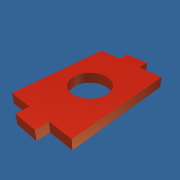
# Autodesk Inventor part: Acrylic_2.2_UpperArmBridge
Saved by Autodesk Inventor 2012 (Build 160160000, 160)
## iProperties
Created: 2014-03-29
Part Number: Acrylic_2.2_UpperArmBridge
Material: Default
Document SubType Name: Modeling
Designer: Admin
Density: 1 g/cm^3
Author: Admin
Autodesk Inventor part; units mm, degrees
ref_plane "YZ Plane" through (0, 0, 0) normal (1, 0, 0) x (0, 1, 0)
ref_plane "XZ Plane" through (0, 0, 0) normal (0, 1, 0) x (-1, 0, 0)
ref_plane "XY Plane" through (0, 0, 0) normal (0, 0, 1) x (1, 0, 0)
sketch "Sketch1" plane through (0, 0, 0) normal (0, 0, 1) x (1, 0, 0)
  line L0 (-10.5, 0) -> (10.5, 0) projected
  line L1 (0, -18.9) -> (0, 18.9) projected
  line L2 (-2.5, -11) -> (-2.5, -13.5)
  line L3 (-2.5, -13.5) -> (2.5, -13.5)
  line L4 (2.5, -13.5) -> (2.5, -11)
  line L5 (-2.5, 11) -> (-2.5, 13.5)
  line L6 (-2.5, 13.5) -> (2.5, 13.5)
  line L7 (2.5, 13.5) -> (2.5, 11)
  line L8 (7.5, 11) -> (7.5, -11)
  line L9 (-7.5, -11) -> (-7.5, 11)
  line L10 (-7.5, 11) -> (-2.5, 11)
  line L11 (2.5, 11) -> (7.5, 11)
  line L12 (7.5, -11) -> (2.5, -11)
  line L13 (-2.5, -11) -> (-7.5, -11)
  circle A0 centre (0, 0) radius 4
  dimension "d7" = 2.5
  dimension "d8" = 2.5
  dimension "d10" = 2.5
  dimension "d11" = 2.5
  dimension "d14" = 22
  dimension "d16" = 7.5
  dimension "d17" = 15
  dimension "d18" = 2.5
  dimension "d19" = 2.5
  dimension "d20" = 8
  constraints: 24 end point, 5 parallel, 4 perpendicular, 2 horizontal, 1 centre point, 1 coincident
  measures "d7" distance between parallel lines of L1 L2
  measures "d8" distance between parallel lines of L4 L1
  measures "d10" distance between parallel lines of L1 L5
  measures "d11" distance between parallel lines of L7 L1
  measures "d14" distance of L8.start L8.end
  measures "d16" distance between parallel lines of L1 L8
  measures "d17" distance of L9.end L8.start
  measures "d18" distance of L3.end L4.end
  measures "d19" distance of L6.end L7.end
  measures "d20" diameter of A0
extrude "Extrusion1" add sketch "Sketch1" along normal blind 2.2 contours L9 L10 L5 L6 L1 A0 L0 | L0 A0 L1 L3 L2 L13 L9 | L1 L6 L7 L11 L8 L0 A0 | A0 L0 L8 L12 L4 L3 L1
equation "\"d16\" = 0.5 * d17"
equation "\"d2\" = 0.5 * d1"
equation "\"d15\" = 0.5 * d14"
equation "\"d1\" = 50"
body "Solid1"
